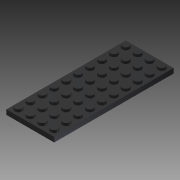
# Autodesk Inventor part: LEGO Plate 4x10
Saved by Autodesk Inventor 2013 (Build 170138000, 138)
## iProperties
Created: 2013-06-01
Part Number: LEGO Plate 4x10
Material: Generic
Document SubType Name: Modeling
Designer: Masta
Density: 1 g/cm^3
Author: Masta
Autodesk Inventor part; units mm, degrees
ref_plane "YZ Plane" through (0, 0, 0) normal (1, 0, 0) x (0, 1, 0)
ref_plane "XZ Plane" through (0, 0, 0) normal (0, 1, 0) x (-1, 0, 0)
ref_plane "XY Plane" through (0, 0, 0) normal (0, 0, 1) x (1, 0, 0)
sketch "Sketch1" plane through (0, 0, 0) normal (0, 0, 1) x (1, 0, 0)
  line L0 (-4, -4) -> (4, -4)
  line L1 (4, -4) -> (4, 4)
  line L2 (4, 4) -> (-4, 4)
  line L3 (-4, 4) -> (-4, -4)
  line L4 (-4, -4) -> (4, 4) construction
  line L5 (4, -4) -> (-4, 4) construction
  circle A0 centre (0, 0) radius 2.4
  dimension "d0" = 8
  dimension "d1" = 8
  dimension "d2" = 4.8
  constraints: 12 end point, 2 midpoint, 2 parallel, 1 centre point, 1 coincident, 1 horizontal, 1 perpendicular
  measures "d0" distance of L2.end L1.end
  measures "d1" distance of L1.end L0.end
  measures "d2" diameter of A0
extrude "Extrusion1" add sketch "Sketch1" along normal blind 3.2 contours L3 L2 L1 L0 | A0
extrude "Extrusion2" add sketch "Sketch1" along normal blind 4.9 contours A0
extrude "Extrusion3" cut sketch "Sketch1" along normal blind 1.7 contours A0
pattern_linear "Rectangular Pattern1" count 10 spacing 8 along (0, 1, 0) count 4 spacing 8 along (1, 0, 0) of "Extrusion1", "Extrusion2", "Extrusion3"
equation "\"d11\" = d0"
equation "\"d24\" = d0"
body "Solid1"
